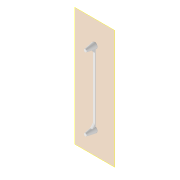
# Autodesk Inventor part: 40_microfluidic_chip_lightsheet_layer1_v0
Saved by Autodesk Inventor 2022 (Build 260153000, 153)
## iProperties
Created: 2021-12-21
Part Number: 40_microfluidic_chip_lightsheet_layer1_v0
Material: Generisch
Document SubType Name: Modeling
Designer: diederichbenedict
Density: 1 g/cm^3
Appearance: Vorgabe
Author: diederichbenedict
Autodesk Inventor part; units mm, degrees
ref_plane "YZ Plane" through (0, 0, 0) normal (1, 0, 0) x (0, 1, 0)
ref_plane "XZ Plane" through (0, 0, 0) normal (0, 1, 0) x (-1, 0, 0)
ref_plane "XY Plane" through (0, 0, 0) normal (0, 0, 1) x (1, 0, 0)
ref_plane "Arbeitsebene1" through (0, 0, 0) normal (0, 0, 1) x (1, 0, 0)
sketch "Skizze1" plane through (0, 0, 0) normal (0, 0, 1) x (1, 0, 0)
  line L0 (-0.75, -25) -> (0.75, -25)
  line L1 (0.75, -25) -> (0.75, 25)
  line L2 (0.75, 25) -> (-0.75, 25)
  line L3 (-0.75, 25) -> (-0.75, -25)
  line L4 (-0.75, -25) -> (0.75, 25) construction
  line L5 (0.75, -25) -> (-0.75, 25) construction
  circle A0 centre (0, 25) radius 2
  circle A1 centre (0, -25) radius 2
  point P0 (0, 0)
  point P1 (0.75, -23.146)
  point P2 (0.75, 23.146)
  point P3 (-0.75, 23.146)
  point P4 (-0.75, -23.146)
  dimension "d0" = 1.5
  dimension "d1" = 50
  dimension "d2" = 4
  dimension "d3" = 4
  constraints: 12 end point, 4 midpoint, 2 centre point, 2 parallel, 1 horizontal, 1 perpendicular
  measures "d0" distance of L2.end L1.end
  measures "d1" distance of L1.end L0.end
  measures "d2" diameter of A0
  measures "d3" diameter of A1
extrude "Extrusion1" add sketch "Skizze1" along normal blind 0.5
sketch "Skizze2" plane through (0, 0, 0.5) normal (0, 0, 1) x (1, 0, 0)
  arc A0 (0.75, 23.146) -> (-0.75, 23.146) centre (0, 25) ccw projected
  arc A1 (-0.75, -23.146) -> (0.75, -23.146) centre (0, -25) ccw projected
  circle A2 centre (0, 25) radius 2
  circle A3 centre (0, -25) radius 2
  point P0 (0, 0)
  point P1 (0.75, -23.146)
  point P2 (-0.75, -23.146)
  point P3 (-0.75, 23.146)
  point P4 (0.75, 23.146)
  constraints: 2 centre point, 2 coincident, 2 concentric
extrude "Extrusion2" add sketch "Skizze2" along normal blind 6 draft -10
chamfer "Fase1" distance 2 angle 45 2 edges at (0, 23, 0.5) (0, -23, 0.5)
